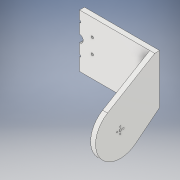
# Autodesk Inventor part: HA004
Saved by Autodesk Inventor 2017 SP1 (Build 210196100, 196)
## iProperties
Created: 2017-06-10
Part Number: HA004
Material: Generic
Document SubType Name: Modeling
Designer: Zach
Density: 1 g/cm^3
Appearance: CR White
Author: Zach
Autodesk Inventor part; units mm, degrees
ref_plane "YZ Plane" through (0, 0, 0) normal (1, 0, 0) x (0, 1, 0)
ref_plane "XZ Plane" through (0, 0, 0) normal (0, 1, 0) x (-1, 0, 0)
sketch "Sketch1" plane through (0, 0, 0) normal (0, 0, 1) x (1, 0, 0)
  line L0 (-152.5, -50) -> (152.5, -50)
  line L1 (152.5, -50) -> (152.5, 50)
  line L2 (152.5, 50) -> (-152.5, 50)
  line L3 (-152.5, 50) -> (-152.5, -50)
  line L4 (-152.5, -50) -> (152.5, 50) construction
  line L5 (152.5, -50) -> (-152.5, 50) construction
  point P0 (0, 0)
  dimension "d0" = 305
  dimension "d1" = 100
  constraints: 12 end point, 2 midpoint, 2 parallel, 1 horizontal, 1 perpendicular
  measures "d0" distance of L2.end L1.end
  measures "d1" distance of L1.end L0.end
extrude "Extrusion1" add sketch "Sketch1" along normal blind 10
sketch "Sketch4" plane through (152.5, -50, 0) normal (1, 0, 0) x (0, 0, -1)
  circle A0 centre (-80, 0) radius 50 construction
  line L0 (0, 0) -> (-10, 0)
  line L1 (0, 0) -> (-48.75, -39.0312)
  line L2 (-10, 0) -> (-10, 100)
  line L3 (-10, 100) -> (-105.6226, 42.9358)
  arc A1 (-105.6226, 42.9358) -> (-48.75, -39.0312) centre (-80, 0) ccw
  line L4 (0, 0) -> (-10, 0)
  line L5 (-10, 100) -> (-10, 0)
  dimension "d8" = 100
  dimension "d20" = 80
  constraints: 12 end point, 4 point on circle, 4 tangent, 3 coincident, 2 centre point, 2 collinear, 1 horizontal alignment
  measures "d8" diameter of A0
  measures "d20" distance of point (0, 0) A0.centre
extrude "Extrusion3" add sketch "Sketch4" against normal blind 305
ref_plane "Work Plane1" through (0, 0, 10) normal (0, 0, 1) x (1, 0, 0)
sketch "Sketch5" plane through (0, 0, 10) normal (0, 0, 1) x (1, 0, 0)
  line L0 (152.5, 50) -> (-152.5, 50) projected
  line L1 (152.5, -100) -> (-152.5, -100) projected
  line L2 (-142.5, 50) -> (142.5, 50)
  line L3 (142.5, 50) -> (142.5, -100)
  line L4 (142.5, -100) -> (-142.5, -100)
  line L5 (-142.5, -100) -> (-142.5, 50)
  line L6 (-152.5, 50) -> (-152.5, -50) projected
  line L7 (152.5, -50) -> (152.5, 50) projected
  point P0 (0, 0)
  dimension "d16" = 10
  dimension "d17" = 10
  constraints: 8 end point, 2 parallel, 2 point on line, 1 horizontal, 1 perpendicular
  measures "d16" distance between parallel lines of L6 L5
  measures "d17" distance between parallel lines of L7 L3
extrude "Extrusion4" cut sketch "Sketch5" along normal through all
sketch "Sketch9" plane through (152.5, -50, 0) normal (1, 0, 0) x (0, 0, -1)
  arc A0 (-105.6226, 42.9358) -> (-48.75, -39.0312) centre (-80, 0) ccw projected
  circle A1 centre (-80, 0) radius 2.5
  point P0 (0, 50)
  dimension "d28" = 5
  constraints: 1 centre point, 1 coincident
  measures "d28" diameter of A1
extrude "Extrusion8" cut sketch "Sketch9" against normal through all
sketch "Sketch11" plane through (0, 0, 10) normal (0, 0, 1) x (1, 0, 0)
  circle A0 centre (0, -30) radius 2.5
  circle A1 centre (25.9808, -15) radius 2.5
  circle A2 centre (25.9808, 15) radius 2.5
  circle A3 centre (0, 30) radius 2.5
  circle A4 centre (-25.9808, 15) radius 2.5
  circle A5 centre (-25.9808, -15) radius 2.5
  circle A6 centre (0, 0) radius 7.5
  dimension "d33" = 5
  dimension "d34" = 30
  dimension "d37" = 360
  dimension "d41" = 15
  constraints: 7 centre point, 1 coincident, 1 vertical alignment, 13 other
  measures "d33" diameter of A0
  measures "d34" distance of A0.centre point (0, 0)
  measures "d41" diameter of A6
extrude "Extrusion10" cut sketch "Sketch11" against normal through all
sketch "Sketch14" plane through (-142.5, -58.0064, 10) normal (1, 0, 0) x (0, 0, -1)
  circle A0 centre (-70, 8.0064) radius 2.5 projected
  circle A1 centre (-70, 14.3564) radius 1.5
  circle A2 centre (-76.35, 8.0064) radius 1.5
  circle A3 centre (-70, 1.6564) radius 1.5
  circle A4 centre (-63.65, 8.0064) radius 1.5
  point P0 (10, 58.0064)
  dimension "d49" = 3
  dimension "d50" = 6.35
  dimension "d53" = 360
  constraints: 4 centre point, 1 vertical alignment, 9 other
  measures "d49" diameter of A1
  measures "d50" distance of A1.centre A0.centre
extrude "Extrusion12" cut sketch "Sketch14" along normal through all both and the other way through all contours A1 | A2 | A3 | A4
sketch "Sketch15" plane through (0, 0, 10) normal (0, 0, 1) x (1, 0, 0)
  line L0 (152.5, 50) -> (-152.5, 50) projected
  line L1 (-152.5, -7.0642) -> (-152.5, -100) projected
  line L2 (0, 50) -> (-152.5, 50)
  line L3 (-152.5, 50) -> (-152.5, -100)
  line L4 (-152.5, -100) -> (0, -100)
  line L5 (0, -100) -> (0, 50)
  point P0 (0, 0)
  point P1 (-152.5, -89.0312)
  constraints: 8 end point, 2 parallel, 1 horizontal, 1 midpoint, 1 perpendicular
extrude "Extrusion13" cut sketch "Sketch15" along normal through all both and the other way through all
body "Solid1"
